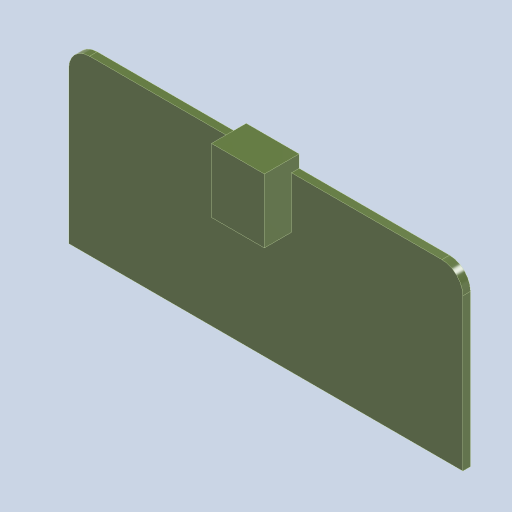
# Autodesk Inventor part: PCB
Saved by Autodesk Inventor 2024.4 (Build 284460000, 460)
## iProperties
Created: 2026-03-16
Part Number: PCB
Material: Generic
Document SubType Name: Modeling
Designer: tooles01
Density: 1 g/cm^3
Appearance: Dark Olive
Author: tooles01
Autodesk Inventor part; units mm, degrees
ref_plane "YZ Plane" through (0, 0, 0) normal (1, 0, 0) x (0, 1, 0)
ref_plane "XZ Plane" through (0, 0, 0) normal (0, 1, 0) x (-1, 0, 0)
ref_plane "XY Plane" through (0, 0, 0) normal (0, 0, 1) x (1, 0, 0)
sketch "Sketch1: PCB" plane through (0, 0, 0) normal (0, 0, 1) x (1, 0, 0)
  line L0 (-22.0554, 53.3935) -> (34.5446, 53.3935)
  line L1 (34.5446, 53.3935) -> (34.5446, 28.5935)
  line L2 (34.5446, 28.5935) -> (-22.0554, 28.5935)
  line L3 (-22.0554, 28.5935) -> (-22.0554, 53.3935)
  line L4 (2.3446, 55.1935) -> (9.9446, 55.1935)
  line L5 (9.9446, 55.1935) -> (9.9446, 45.9935)
  line L6 (9.9446, 45.9935) -> (2.3446, 45.9935)
  line L7 (2.3446, 45.9935) -> (2.3446, 55.1935)
  point P0 (0, 0)
  dimension "d0" = 56.6
  dimension "d1" = 24.8
  dimension "d2" = 7.6
  dimension "d4" = 9.2
  dimension "d7" = 1.8
  dimension "d13" = 32
  constraints: 16 end point, 4 perpendicular, 2 horizontal, 1 other
  measures "d0" distance of L0.start L0.end
  measures "d1" distance of L2.end L0.start
  measures "d2" distance of L5.end L6.end
  measures "d4" distance of L6.end L4.start
  measures "d7" distance between parallel lines of L0 L4
  measures "d13" distance between parallel lines of L3 L5
extrude "Extrusion1" add sketch "Sketch1: PCB" along normal blind 1.1 contours L0 L7 L6 L5 L1 L2 L3 | L0 L5 L6 L7
extrude "Extrusion2" add sketch "Sketch1: PCB" along normal blind 5 contours L7 L4 L5 L0 | L0 L5 L6 L7
fillet "Fillet1" radius 3 2 edges at (-22.0554, 53.3935, 0.55) (34.5446, 53.3935, 0.55)
body "Solid1"
